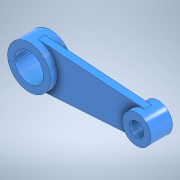
# Autodesk Inventor part: Manipulo
Saved by Autodesk Inventor 2021 (Build 250183000, 183)
## iProperties
Created: 2021-04-08
Part Number: Manipulo
Material: Genérico
Document SubType Name: Modeling
Designer: rubia
Density: 1 g/cm^3
Appearance: Ciano
Author: rubia
Autodesk Inventor part; units mm, degrees
ref_plane "YZ Plane" through (0, 0, 0) normal (1, 0, 0) x (0, 1, 0)
ref_plane "XZ Plane" through (0, 0, 0) normal (0, 1, 0) x (-1, 0, 0)
ref_plane "XY Plane" through (0, 0, 0) normal (0, 0, 1) x (1, 0, 0)
sketch "Esboço1" plane through (0, 0, 0) normal (0, 0, 1) x (1, 0, 0)
  circle A0 centre (0, 0) radius 8
  arc A1 (0.8, 11.9733) -> (0.8, -11.9733) centre (0, 0) ccw
  arc A2 (60.5333, -7.9822) -> (60.5333, 7.9822) centre (60, 0) ccw
  circle A3 centre (60, 0) radius 4
  line L0 (0.8, 11.9733) -> (60.5333, 7.9822)
  line L1 (0, 0) -> (60, 0) construction
  line L2 (0.8, -11.9733) -> (60.5333, -7.9822)
  point P0 (-9.6543, 12.6718)
  point P1 (71.6078, 7.2423)
  point P2 (-9.6543, -12.6718)
  point P3 (71.6078, -7.2423)
  dimension "d0" = 16
  dimension "d1" = 24
  dimension "d2" = 16
  dimension "d3" = 8
  dimension "d4" = 60
  constraints: 6 end point, 4 centre point, 4 point on circle, 3 coincident, 2 symmetric about line, 2 tangent, 1 horizontal, 1 horizontal alignment
  measures "d0" diameter of A0
  measures "d1" diameter of A1
  measures "d2" diameter of A2
  measures "d3" diameter of A3
  measures "d4" distance of point (0, 0) A2.centre
extrude "Extrusão1" add sketch "Esboço1" along normal mid plane 4
sketch "Esboço2" plane through (0, 0, 0) normal (0, 0, 1) x (1, 0, 0)
  circle A0 centre (0, 0) radius 8
  circle A1 centre (0, 0) radius 12
  circle A2 centre (60, 0) radius 4 projected
  circle A3 centre (60, 0) radius 4
  line L0 (60.5333, 7.9822) -> (0.8, 11.9733) projected
  circle A4 centre (60, 0) radius 8
  constraints: 4 coincident, 2 centre point, 5 other
extrude "Extrusão2" add sketch "Esboço2" along normal mid plane 12
sketch "Esboço3" plane through (0, 0, 6) normal (0, 0, 1) x (1, 0, 0)
  circle A0 centre (0, 0) radius 8 projected
  line L0 (-8, 0) -> (-6.8, 0)
  line L1 (-6.8, 0) -> (-6.8, 0.6)
  line L2 (-6.8, 0.6) -> (-8, 0.6)
  line L3 (-8, 0.6) -> (-8, 0)
  line L4 (-8, 0) -> (-6.8, 0)
  line L5 (-6.8, 0) -> (-6.8, -0.6)
  line L6 (-6.8, -0.6) -> (-8, -0.6)
  line L7 (-8, -0.6) -> (-8, 0)
  dimension "d9" = 1.2
  dimension "d10" = 0.6
  dimension "d11" = 1.2
  dimension "d12" = 0.6
  constraints: 16 end point, 4 parallel, 2 horizontal, 2 perpendicular, 1 horizontal alignment, 1 other
  measures "d9" distance of L2.end L1.end
  measures "d10" distance of L1.end L0.end
  measures "d11" distance of L5.end L6.end
  measures "d12" distance of L4.end L5.end
extrude "Extrusão3" add sketch "Esboço3" against normal blind 12 contours L2 L1 L0 A0 | A0 L3 L2 | L6 L7 A0 | A0 L0 L5 L6
